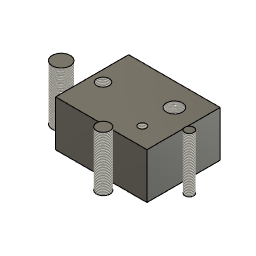
sketch constraints (Autodesk Fusion 360 design; units mm, degrees)
Autodesk Fusion 360 part; units mm, degrees
sketch "Sketch1" plane through (0, 0, 0) normal (0, 1, 0) x (1, 0, 0)
  line L0 (50, -40) -> (-50, -40)
  line L1 (-50, -40) -> (-50, 40)
  line L2 (-50, 40) -> (50, 40)
  line L3 (50, 40) -> (50, -40)
  line L4 (50, -40) -> (-50, 40) construction
  line L5 (-50, -40) -> (50, 40) construction
  dimension "d1" = 80
  dimension "d2" = 100
  constraint perpendicular L0 L1
  constraint parallel L0 L2
  constraint parallel L1 L3
  constraint horizontal L0
  constraint coincident L4 origin
  constraint coincident L5 origin
  measures "d1" distance of L0.end L1.end
  measures "d2" distance of L1.end L2.end
extrude "Extrude1" add sketch "Sketch1" along normal blind 50 makes body 1
ref_plane "WorkPlane1" through (0, 10, 0) normal (0, 1, 0) x (0, 0, 1)
sketch "Hole" plane through (0, 10, 0) normal (0, 1, 0) x (1, 0, 0)
  circle A0 centre (25, -20) radius 5
  circle A1 centre (-38, 0) radius 7.5
  circle A2 centre (25, 15) radius 10
  line L0 (-50, 40) -> (50, 40)
  line L1 (50, 40) -> (50, -40)
  line L2 (50, -40) -> (-50, -40)
  line L3 (-50, -40) -> (-50, 40)
  line L4 (50, -40) -> (-50, 40)
  dimension "d6" = 10
  dimension "d7" = 15
  dimension "d8" = 20
  dimension "d30" = 25
  dimension "d31" = 25
  dimension "d32" = 20
  dimension "d33" = 12
  constraint horizontal origin A1.centre
  constraint coincident A0.centre L4
  measures "d6" diameter of A0
  measures "d7" diameter of A1
  measures "d8" diameter of A2
  measures "d30" distance of A2.centre L0
  measures "d31" distance of A2.centre L1
  measures "d32" distance of A0.centre L2
  measures "d33" distance of A1.centre L3
extrude "Extrude5" cut sketch "Hole" along normal blind 60 contours A2 bodies 1
extrude "Extrude6" cut sketch "Hole" along normal blind 60 contours A0 L4 | A0 L4 bodies 1
extrude "Extrude7" cut sketch "Hole" along normal blind 60 contours A1 bodies 1
sketch "Rod" plane through (0, 10, 0) normal (0, 1, 0) x (1, 0, 0)
  circle A0 centre (74.3742, -18.093) radius 5
  circle A1 centre (24.417, -62.1821) radius 7.5
  circle A2 centre (-61.2458, -22.5024) radius 10
  dimension "d21" = 10
  dimension "d22" = 15
  dimension "d23" = 20
  measures "d21" diameter of A0
  measures "d22" diameter of A1
  measures "d23" diameter of A2
extrude "Extrude8" add sketch "Rod" along normal blind 60 separate body contours A0 makes body 2
extrude "Extrude9" add sketch "Rod" along normal blind 60 separate body contours A1 makes body 3
extrude "Extrude10" add sketch "Rod" along normal blind 60 separate body contours A2 makes body 4
copy_body "Body->Comp1" bodies 1 removing the originals makes body 5 in component "Block"
copy_body "Body->Comp2" bodies 2 removing the originals makes body 6 in component "Rod 1"
copy_body "Body->Comp3" bodies 3 removing the originals makes body 7 in component "Rod 2"
copy_body "Body->Comp4" bodies 4 removing the originals makes body 8 in component "Rod 3"
thread "Thread1" "ISO Metric profile 15.0 M15x1.5 6H" major diameter 15.2033 minor diameter 13.5262 pitch 1.5 angle 60 resizes the face on face at (-30.5373, 36.6667, -0.7468) on bodies 5 in component "Block"
thread "Thread2" "ISO Metric profile 20.0 M20x2.5 6H" major diameter 20.2925 minor diameter 17.519 pitch 2.5 angle 60 resizes the face on face at (34.9876, 23.3333, -15.4985) on bodies 5 in component "Block"
thread "Thread3" "ISO Metric profile 10.0 M10x1.5 6H" major diameter 10.198 minor diameter 8.526 pitch 1.5 angle 60 resizes the face on face at (29.9938, 23.3333, 19.7508) on bodies 5 in component "Block"
thread "Thread1'" "ISO Metric profile 10.0 M10x1.5 6g" major diameter 9.85 minor diameter 8.141 pitch 1.5 angle 60 resizes the face on face at (79.3494, 50, 18.5909) on bodies 6 in component "Rod 1"
thread "Thread1''" "ISO Metric profile 15.0 M15x1.5 6g" major diameter 14.85 minor diameter 13.1369 pitch 1.5 angle 60 resizes the face on face at (31.8798, 50, 62.9289) on bodies 7 in component "Rod 2"
thread "Thread1'''" "ISO Metric profile 20.0 M20x2.5 6g" major diameter 19.7905 minor diameter 16.938 pitch 2.5 angle 60 resizes the face on face at (-51.2955, 50, 23.4981) on bodies 8 in component "Rod 3"
component "Block" placed x (1, 0, 0) y (0, 1, 0) z (0, 0, 1) at (0, 0, 0)
component "Rod 1" placed x (1, 0, 0) y (0, 1, 0) z (0, 0, 1) at (0, 0, 0)
component "Rod 2" placed x (1, 0, 0) y (0, 1, 0) z (0, 0, 1) at (0, 0, 0)
component "Rod 3" placed x (1, 0, 0) y (0, 1, 0) z (0, 0, 1) at (0, 0, 0)
